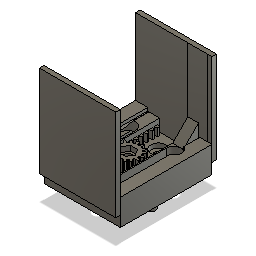
Spool Saver (Autodesk Fusion 360 design; units mm, degrees)
description: Spur Gear; Module: 1.000000; Num Teeth: 16; Pressure Angle: 20.000000; Backlash: 0.05 mm
Autodesk Fusion 360 part; units mm, degrees
(part 1 of 5)
sketch "Side Profile" plane through (0, 0, 0) normal (0, 0, 1) x (1, 0, 0)
  line L0 (0, 0) -> (25, 0)
  line L1 (25, 7) -> (3, 7)
  line L2 (8, 17.2) -> (0, 17.2)
  line L3 (0, 17.2) -> (0, 0)
  line L4 (8, 17.2) -> (8, 15.2)
  line L5 (3, 7) -> (3, 8.0593)
  line L6 (3, 8.0593) -> (8, 15.2)
  line L7 (50, 17.2) -> (50, 0)
  line L8 (50, 0) -> (25, 0)
  line L9 (47, 7) -> (47, 8.0593)
  line L10 (42, 17.2) -> (50, 17.2)
  line L11 (47, 8.0593) -> (42, 15.2)
  line L12 (25, 7) -> (47, 7)
  line L13 (42, 17.2) -> (42, 15.2)
  point P0 (50, 0)
  dimension "d2" = 7
  dimension "d3" = 17.2
  dimension "d4" = 8
  dimension "d5" = 2
  dimension "d8" = 22
  dimension "d9" = 145
  constraint coincident L0.start L3.end
  constraint horizontal L0
  constraint perpendicular L0 L3
  constraint perpendicular L2 L4
  constraint perpendicular L1 L5
  measures "d2" distance of L0.end L1.start
  measures "d3" distance of L0.start L2.end
  measures "d4" distance of L2.start L2.end
  measures "d5" distance of L2.start L4.end
  measures "d8" distance of L1.start L1.end
  measures "d9" angle of L4 L6
extrude "Extrude1" add sketch "Side Profile" along normal blind 60 makes body 1
sketch "Base Top" plane through (0, 7, 0) normal (0, 1, 0) x (-1, 0, 0)
  line L0 (-47, 0) -> (-3, 0)
  line L1 (-3, 0) -> (-3, 60)
  line L2 (-3, 60) -> (-47, 60)
  circle A0 centre (-25, 30) radius 4.475
  circle A1 centre (-25, 30) radius 2.6
  line L3 (0, 0) -> (0, 60)
  line L4 (-50, 0) -> (-50, 60)
  line L5 (0, 30) -> (-50, 30) construction
  circle A2 centre (-40, 15) radius 2.45
  line L6 (-3, 0) -> (-47, 0)
  line L7 (-50, 0) -> (-50, 60)
  circle A3 centre (-10, 45) radius 2.45
  circle A4 centre (-40, 15) radius 5
  circle A5 centre (-10, 45) radius 5
  line L8 (-47, 60) -> (-47, 0)
  line L9 (-47, 0) -> (-3, 0)
  line L10 (-3, 0) -> (-3, 60)
  line L11 (-3, 60) -> (-47, 60)
  line L12 (-47, 60) -> (-47, 0)
  line L13 (-37.55, 15) -> (-37.55, 3)
  line L14 (-42, 0) -> (-42, 60)
  line L15 (-42.45, 15) -> (-42.45, 3)
  line L16 (-37.55, 3) -> (-42.45, 3)
  line L17 (-12.45, 45) -> (-12.45, 57)
  line L18 (-8, 0) -> (-8, 60)
  line L19 (-7.55, 45) -> (-7.55, 57)
  line L20 (-12.45, 57) -> (-7.55, 57)
  circle A6 centre (-25, 10) radius 2.6
  circle A7 centre (-25, 10) radius 5
  line L21 (0, 0) -> (0, 60)
  circle A8 centre (-25, 50) radius 2.6
  circle A9 centre (-25, 50) radius 5
  dimension "d14" = 8.95
  dimension "d15" = 5.2
  dimension "d20" = 4.9
  dimension "d21" = 15
  dimension "d22" = 10
  dimension "d24" = 10
  dimension "d25" = 10
  dimension "d26" = 15
  dimension "d46" = 12
  dimension "d115" = 5.2
  dimension "d116" = 10
  dimension "d117" = 10
  dimension "d118" = 25
  constraint coincident A0.centre A1.centre
  constraint midpoint L3 L5.start
  constraint midpoint L4 L5.end
  constraint equal A2 A3
  constraint concentric A2 A4
  constraint concentric A3 A5
  constraint equal A4 A5
  constraint vertical L13
  constraint parallel L14 L15
  constraint equal L13 L15
  constraint tangent A2 L13
  constraint tangent A2 L15
  constraint coincident A2 L13.start
  constraint coincident A2 L15.start
  constraint coincident A3 L17.start
  constraint coincident A3 L19.start
  constraint parallel L18 L19
  constraint equal L13 L17
  constraint equal L15 L19
  constraint equal L16 L20
  constraint concentric A6 A7
  constraint symmetric L5 A6 A8
  constraint symmetric L5 A7 A9
  measures "d14" diameter of A0
  measures "d15" diameter of A1
  measures "d20" diameter of A2
  measures "d21" distance of A2.centre L6
  measures "d22" distance of A2.centre L7
  measures "d24" diameter of A4
  measures "d25" distance of L3 A3.centre
  measures "d26" distance of L2 A3.centre
  measures "d46" distance of L13.start L13.end
  measures "d115" diameter of A6
  measures "d116" diameter of A7
  measures "d117" distance of L6 A6.centre
  measures "d118" distance of A6.centre L21
extrude "Extrude4" cut sketch "Base Top" against normal up to surface (7 mm away) contours A3 L18 | A3 L18 | A2 L14 | A2 L14 | A1 bodies 1
extrude "Extrude5" add sketch "Base Top" along normal blind 2.5 contours A0 bodies 1
sketch "Sketch1" plane through (0, 0, 0) normal (0, 0, 1) x (1, 0, 0) in component "Spur Gear (16 teeth)"
  circle A0 centre (0, 0) radius 6.7492
  circle A1 centre (0, 0) radius 2.5
extrude "Extrude1'" add sketch "Sketch1" along normal blind 5 separate body makes body 2 in component "Spur Gear (16 teeth)"
sketch "Sketch2" plane through (0, 0, 0) normal (0, 0, 1) x (1, 0, 0) in component "Spur Gear (16 teeth)"
  spline S0 degree 5 poles (7.4708, -0.8366) (7.4752, -0.8371) (7.4838, -0.8379) (7.4968, -0.8388) (7.5141, -0.8393) (7.5358, -0.8389) (7.5576, -0.8379) (7.5793, -0.8364) (7.6012, -0.8347) (7.623, -0.8328) (7.6449, -0.8308) (7.6667, -0.8285) (7.6886, -0.826) (7.7105, -0.8231) (7.7325, -0.8199) (7.7544, -0.8163) (7.7763, -0.8125) (7.7983, -0.8084) (7.8202, -0.8042) (7.8422, -0.7997) (7.8641, -0.7951) (7.8861, -0.7903) (7.9081, -0.7852) (7.93, -0.78) (7.952, -0.7745) (7.974, -0.7688) (7.9959, -0.763) (8.0179, -0.7569) (8.0399, -0.7506) (8.0618, -0.7442) (8.0838, -0.7376) (8.1057, -0.7308) (8.1277, -0.7239) (8.1496, -0.7168) (8.1716, -0.7095) (8.1935, -0.702) (8.2154, -0.6944) (8.2373, -0.6865) (8.2592, -0.6786) (8.2811, -0.6704) (8.303, -0.6622) (8.3248, -0.6537) (8.3467, -0.6451) (8.3685, -0.6363) (8.3904, -0.6274) (8.4122, -0.6183) (8.434, -0.6091) (8.4558, -0.5997) (8.4776, -0.5902) (8.4993, -0.5805) (8.5211, -0.5707) (8.5428, -0.5607) (8.5645, -0.5506) (8.5862, -0.5403) (8.6079, -0.5299) (8.6295, -0.5193) (8.6511, -0.5086) (8.6728, -0.4978) (8.6944, -0.4868) (8.7159, -0.4757) (8.7375, -0.4644) (8.759, -0.453) (8.7805, -0.4415) (8.802, -0.4298) (8.8235, -0.418) (8.8449, -0.4061) (8.8664, -0.394) (8.8878, -0.3818) (8.9091, -0.3695) (8.9305, -0.357) (8.9518, -0.3444) (8.9688, -0.3342) (8.9816, -0.3265) (8.9901, -0.3213) (8.9944, -0.3187) knots 0 0 0 0 0 0 0.01428571 0.02857143 0.04285714 0.05714286 0.07142857 0.08571429 0.1 0.11428571 0.12857143 0.14285714 0.15714286 0.17142857 0.18571429 0.2 0.21428571 0.22857143 0.24285714 0.25714286 0.27142857 0.28571429 0.3 0.31428571 0.32857143 0.34285714 0.35714286 0.37142857 0.38571429 0.4 0.41428571 0.42857143 0.44285714 0.45714286 0.47142857 0.48571429 0.5 0.51428571 0.52857143 0.54285714 0.55714286 0.57142857 0.58571429 0.6 0.61428571 0.62857143 0.64285714 0.65714286 0.67142857 0.68571429 0.7 0.71428571 0.72857143 0.74285714 0.75714286 0.77142857 0.78571429 0.8 0.81428571 0.82857143 0.84285714 0.85714286 0.87142857 0.88571429 0.9 0.91428571 0.92857143 0.94285714 0.95714286 0.97142857 0.98571429 1 1 1 1 1 1
  spline S1 degree 5 poles (7.4708, 0.8366) (7.4752, 0.8371) (7.4838, 0.8379) (7.4968, 0.8388) (7.5141, 0.8393) (7.5358, 0.8389) (7.5576, 0.8379) (7.5793, 0.8364) (7.6012, 0.8347) (7.623, 0.8328) (7.6449, 0.8308) (7.6667, 0.8285) (7.6886, 0.826) (7.7105, 0.8231) (7.7325, 0.8199) (7.7544, 0.8163) (7.7763, 0.8125) (7.7983, 0.8084) (7.8202, 0.8042) (7.8422, 0.7997) (7.8641, 0.7951) (7.8861, 0.7903) (7.9081, 0.7852) (7.93, 0.78) (7.952, 0.7745) (7.974, 0.7688) (7.9959, 0.763) (8.0179, 0.7569) (8.0399, 0.7506) (8.0618, 0.7442) (8.0838, 0.7376) (8.1057, 0.7308) (8.1277, 0.7239) (8.1496, 0.7168) (8.1716, 0.7095) (8.1935, 0.702) (8.2154, 0.6944) (8.2373, 0.6865) (8.2592, 0.6786) (8.2811, 0.6704) (8.303, 0.6622) (8.3248, 0.6537) (8.3467, 0.6451) (8.3685, 0.6363) (8.3904, 0.6274) (8.4122, 0.6183) (8.434, 0.6091) (8.4558, 0.5997) (8.4776, 0.5902) (8.4993, 0.5805) (8.5211, 0.5707) (8.5428, 0.5607) (8.5645, 0.5506) (8.5862, 0.5403) (8.6079, 0.5299) (8.6295, 0.5193) (8.6511, 0.5086) (8.6728, 0.4978) (8.6944, 0.4868) (8.7159, 0.4757) (8.7375, 0.4644) (8.759, 0.453) (8.7805, 0.4415) (8.802, 0.4298) (8.8235, 0.418) (8.8449, 0.4061) (8.8664, 0.394) (8.8878, 0.3818) (8.9091, 0.3695) (8.9305, 0.357) (8.9518, 0.3444) (8.9688, 0.3342) (8.9816, 0.3265) (8.9901, 0.3213) (8.9944, 0.3187) knots 0 0 0 0 0 0 0.01428571 0.02857143 0.04285714 0.05714286 0.07142857 0.08571429 0.1 0.11428571 0.12857143 0.14285714 0.15714286 0.17142857 0.18571429 0.2 0.21428571 0.22857143 0.24285714 0.25714286 0.27142857 0.28571429 0.3 0.31428571 0.32857143 0.34285714 0.35714286 0.37142857 0.38571429 0.4 0.41428571 0.42857143 0.44285714 0.45714286 0.47142857 0.48571429 0.5 0.51428571 0.52857143 0.54285714 0.55714286 0.57142857 0.58571429 0.6 0.61428571 0.62857143 0.64285714 0.65714286 0.67142857 0.68571429 0.7 0.71428571 0.72857143 0.74285714 0.75714286 0.77142857 0.78571429 0.8 0.81428571 0.82857143 0.84285714 0.85714286 0.87142857 0.88571429 0.9 0.91428571 0.92857143 0.94285714 0.95714286 0.97142857 0.98571429 1 1 1 1 1 1
  arc A0 (8.9944, -0.3187) -> (8.9944, 0.3187) centre (0, 0) ccw
  line L0 (6.6973, -0.7511) -> (7.4708, -0.8366)
  line L1 (6.6973, 0.7511) -> (7.4708, 0.8366)
  line L2 (6.6973, -0.7511) -> (6.6973, 0.7511)
  point P0 (7.5774, -0.8365)
  point P1 (7.685, -0.8263)
  point P2 (7.7933, -0.8093)
  point P3 (7.902, -0.7866)
  point P4 (8.0111, -0.7587)
  point P5 (8.1205, -0.7262)
  point P6 (8.23, -0.6891)
  point P7 (8.3395, -0.6479)
  point P8 (8.4491, -0.6026)
  point P9 (8.5586, -0.5533)
  point P10 (8.6679, -0.5002)
  point P11 (8.777, -0.4434)
  point P12 (8.8859, -0.3828)
  point P13 (7.5774, 0.8365)
  point P14 (7.685, 0.8263)
  point P15 (7.7933, 0.8093)
  point P16 (7.902, 0.7866)
  point P17 (8.0111, 0.7587)
  point P18 (8.1205, 0.7262)
  point P19 (8.23, 0.6891)
  point P20 (8.3395, 0.6479)
  point P21 (8.4491, 0.6026)
  point P22 (8.5586, 0.5533)
  point P23 (8.6679, 0.5002)
  point P24 (8.777, 0.4434)
  point P25 (8.8859, 0.3828)
extrude "Extrude2" add sketch "Sketch2" along normal blind 5 bodies 2 in component "Spur Gear (16 teeth)"
fillet "Fillet1" radius 0.5 2 edges at (6.7072, -0.7522, 2.5) (6.7072, 0.7522, 2.5) on bodies 2 in component "Spur Gear (16 teeth)"
pattern_circular "C-Pattern1" count 16 over 360 about axis through (0, 0, 0) along (0, 0, 1) of "Extrude2", "Fillet1" in component "Spur Gear (16 teeth)"
sketch "Sketch3" plane through (0, 0, 0) normal (0, 0, 1) x (1, 0, 0) in component "Spur Gear (16 teeth)"
  circle A0 centre (0, 0) radius 8 construction
move_body "Move1" bodies 2 to x (1, 0, 0) y (0, 1, 0) z (0, 0, 1) at (25, 7, 30) in component "Spur Gear (16 teeth)"
move_body "Move2" bodies 2 to x (1, 0, 0) y (0, 0, -1) z (0, 1, 0) at (0, -23, 37) in component "Spur Gear (16 teeth)"
move_body "Move3" bodies 2 to x (0.980785, 0, -0.19509) y (0, 1, 0) z (0.19509, 0, 0.980785) at (-5.3723, 0, 5.4537) in component "Spur Gear (16 teeth)"
cylinder "CylinderPrimitive1" add diameter 5 height -2.5 placed x (1, 0, 0) y (0, 0, -1) z (0, 1, 0) at (25, 12, 30) bodies 2 in component "Spur Gear (16 teeth)"
extrude "Extrude3" add 1 faces at (22.1207, 12, 28.6457) along direction (0, 1, 0) blind 4 on bodies 2 bodies 2 in component "Spur Gear (16 teeth)"
sketch "Nut and Hole" plane through (0, 16, 0) normal (0, 1, 0) x (-1, 0, 0) in component "Spur Gear (16 teeth)"
  arc A0 (-31.7484, 30.1063) -> (-31.7484, 29.8937) centre (-25, 30) ccw
  arc A1 (-32.2052, 29.3877) -> (-31.7484, 29.8937) centre (-32.2483, 29.8858) ccw
  line L0 (-32.2052, 29.3877) -> (-32.4905, 29.363)
  spline S0 degree 5 poles (-32.4905, 29.363) (-32.4948, 29.3627) (-32.5035, 29.3618) (-32.5163, 29.3601) (-32.5334, 29.3572) (-32.5547, 29.3527) (-32.5758, 29.3474) (-32.5969, 29.3417) (-32.618, 29.3358) (-32.639, 29.3297) (-32.6601, 29.3234) (-32.6811, 29.3169) (-32.702, 29.3101) (-32.723, 29.303) (-32.7438, 29.2956) (-32.7646, 29.2878) (-32.7854, 29.2798) (-32.8061, 29.2715) (-32.8269, 29.2631) (-32.8475, 29.2544) (-32.8682, 29.2456) (-32.8888, 29.2366) (-32.9093, 29.2274) (-32.9298, 29.2179) (-32.9503, 29.2083) (-32.9707, 29.1984) (-32.9911, 29.1884) (-33.0115, 29.1781) (-33.0318, 29.1677) (-33.0521, 29.1571) (-33.0724, 29.1464) (-33.0926, 29.1355) (-33.1127, 29.1244) (-33.1329, 29.1131) (-33.1529, 29.1016) (-33.173, 29.09) (-33.193, 29.0783) (-33.213, 29.0663) (-33.2329, 29.0542) (-33.2528, 29.042) (-33.2726, 29.0296) (-33.2924, 29.017) (-33.3122, 29.0043) (-33.3319, 28.9915) (-33.3515, 28.9785) (-33.3712, 28.9653) (-33.3908, 28.952) (-33.4103, 28.9385) (-33.4298, 28.925) (-33.4492, 28.9112) (-33.4687, 28.8973) (-33.488, 28.8833) (-33.5073, 28.8691) (-33.5266, 28.8548) (-33.5458, 28.8404) (-33.565, 28.8258) (-33.5841, 28.8111) (-33.6032, 28.7963) (-33.6223, 28.7813) (-33.6413, 28.7662) (-33.6602, 28.7509) (-33.6791, 28.7355) (-33.698, 28.72) (-33.7168, 28.7044) (-33.7355, 28.6886) (-33.7542, 28.6727) (-33.7729, 28.6567) (-33.7915, 28.6405) (-33.81, 28.6243) (-33.8285, 28.6079) (-33.847, 28.5913) (-33.8617, 28.578) (-33.8727, 28.568) (-33.88, 28.5613) (-33.8837, 28.5579) knots 0 0 0 0 0 0 0.01428571 0.02857143 0.04285714 0.05714286 0.07142857 0.08571429 0.1 0.11428571 0.12857143 0.14285714 0.15714286 0.17142857 0.18571429 0.2 0.21428571 0.22857143 0.24285714 0.25714286 0.27142857 0.28571429 0.3 0.31428571 0.32857143 0.34285714 0.35714286 0.37142857 0.38571429 0.4 0.41428571 0.42857143 0.44285714 0.45714286 0.47142857 0.48571429 0.5 0.51428571 0.52857143 0.54285714 0.55714286 0.57142857 0.58571429 0.6 0.61428571 0.62857143 0.64285714 0.65714286 0.67142857 0.68571429 0.7 0.71428571 0.72857143 0.74285714 0.75714286 0.77142857 0.78571429 0.8 0.81428571 0.82857143 0.84285714 0.85714286 0.87142857 0.88571429 0.9 0.91428571 0.92857143 0.94285714 0.95714286 0.97142857 0.98571429 1 1 1 1 1 1
  arc A2 (-33.8837, 28.5579) -> (-33.7594, 27.9327) centre (-25, 30) ccw
  spline S1 degree 5 poles (-33.7594, 27.9327) (-33.7547, 27.931) (-33.7453, 27.9276) (-33.7313, 27.9225) (-33.7126, 27.9158) (-33.6892, 27.9076) (-33.6659, 27.8996) (-33.6425, 27.8916) (-33.6191, 27.8838) (-33.5958, 27.8762) (-33.5724, 27.8686) (-33.549, 27.8612) (-33.5257, 27.854) (-33.5023, 27.8469) (-33.479, 27.8399) (-33.4557, 27.833) (-33.4323, 27.8264) (-33.409, 27.8198) (-33.3857, 27.8134) (-33.3624, 27.8071) (-33.3391, 27.801) (-33.3158, 27.795) (-33.2925, 27.7892) (-33.2692, 27.7835) (-33.246, 27.7779) (-33.2227, 27.7725) (-33.1995, 27.7673) (-33.1763, 27.7622) (-33.1531, 27.7572) (-33.1299, 27.7524) (-33.1067, 27.7478) (-33.0836, 27.7433) (-33.0605, 27.7389) (-33.0373, 27.7348) (-33.0142, 27.7307) (-32.9912, 27.7269) (-32.9681, 27.7232) (-32.9451, 27.7196) (-32.9221, 27.7162) (-32.8991, 27.713) (-32.8761, 27.71) (-32.8532, 27.7071) (-32.8303, 27.7044) (-32.8074, 27.7018) (-32.7846, 27.6995) (-32.7617, 27.6973) (-32.7389, 27.6953) (-32.7162, 27.6934) (-32.6935, 27.6918) (-32.6708, 27.6903) (-32.6481, 27.689) (-32.6255, 27.6879) (-32.6029, 27.6871) (-32.5804, 27.6864) (-32.5579, 27.6859) (-32.5355, 27.6857) (-32.5131, 27.6856) (-32.4907, 27.6857) (-32.4684, 27.686) (-32.4461, 27.6866) (-32.4239, 27.6874) (-32.4018, 27.6885) (-32.3798, 27.6899) (-32.3578, 27.6917) (-32.3359, 27.6937) (-32.3141, 27.696) (-32.2923, 27.6984) (-32.2705, 27.701) (-32.2489, 27.7038) (-32.2273, 27.707) (-32.206, 27.7109) (-32.1891, 27.7148) (-32.1765, 27.7182) (-32.1682, 27.7207) (-32.1641, 27.722) knots -1 -1 -1 -1 -1 -1 -0.98571429 -0.97142857 -0.95714286 -0.94285714 -0.92857143 -0.91428571 -0.9 -0.88571429 -0.87142857 -0.85714286 -0.84285714 -0.82857143 -0.81428571 -0.8 -0.78571429 -0.77142857 -0.75714286 -0.74285714 -0.72857143 -0.71428571 -0.7 -0.68571429 -0.67142857 -0.65714286 -0.64285714 -0.62857143 -0.61428571 -0.6 -0.58571429 -0.57142857 -0.55714286 -0.54285714 -0.52857143 -0.51428571 -0.5 -0.48571429 -0.47142857 -0.45714286 -0.44285714 -0.42857143 -0.41428571 -0.4 -0.38571429 -0.37142857 -0.35714286 -0.34285714 -0.32857143 -0.31428571 -0.3 -0.28571429 -0.27142857 -0.25714286 -0.24285714 -0.22857143 -0.21428571 -0.2 -0.18571429 -0.17142857 -0.15714286 -0.14285714 -0.12857143 -0.11428571 -0.1 -0.08571429 -0.07142857 -0.05714286 -0.04285714 -0.02857143 -0.01428571 0 0 0 0 0 0
  line L1 (-32.1641, 27.722) -> (-31.8911, 27.8084)
  arc A3 (-31.2753, 27.5157) -> (-31.8911, 27.8084) centre (-31.7402, 27.3317) ccw
  arc A4 (-31.2753, 27.5157) -> (-31.194, 27.3193) centre (-25, 30) ccw
  arc A5 (-31.4224, 26.677) -> (-31.194, 27.3193) centre (-31.6529, 27.1207) ccw
  line L2 (-31.4224, 26.677) -> (-31.6766, 26.545)
  spline S2 degree 5 poles (-31.6766, 26.545) (-31.6804, 26.543) (-31.6881, 26.5389) (-31.6993, 26.5325) (-31.714, 26.5232) (-31.7319, 26.5109) (-31.7494, 26.4979) (-31.7667, 26.4846) (-31.7839, 26.4711) (-31.801, 26.4574) (-31.818, 26.4435) (-31.835, 26.4295) (-31.8518, 26.4152) (-31.8684, 26.4006) (-31.8848, 26.3858) (-31.9011, 26.3706) (-31.9172, 26.3553) (-31.9332, 26.3397) (-31.9491, 26.324) (-31.9649, 26.3081) (-31.9805, 26.292) (-31.9961, 26.2758) (-32.0116, 26.2594) (-32.0269, 26.2428) (-32.0421, 26.2261) (-32.0573, 26.2092) (-32.0723, 26.1921) (-32.0872, 26.1748) (-32.1019, 26.1574) (-32.1166, 26.1399) (-32.1312, 26.1222) (-32.1457, 26.1044) (-32.1601, 26.0864) (-32.1744, 26.0683) (-32.1886, 26.05) (-32.2026, 26.0316) (-32.2166, 26.0131) (-32.2305, 25.9944) (-32.2443, 25.9756) (-32.258, 25.9567) (-32.2715, 25.9377) (-32.285, 25.9185) (-32.2984, 25.8992) (-32.3117, 25.8798) (-32.3249, 25.8602) (-32.338, 25.8406) (-32.351, 25.8208) (-32.3639, 25.8009) (-32.3767, 25.7808) (-32.3894, 25.7607) (-32.402, 25.7405) (-32.4146, 25.7201) (-32.427, 25.6996) (-32.4393, 25.679) (-32.4516, 25.6583) (-32.4637, 25.6375) (-32.4757, 25.6166) (-32.4877, 25.5956) (-32.4996, 25.5744) (-32.5113, 25.5532) (-32.523, 25.5319) (-32.5346, 25.5104) (-32.546, 25.4889) (-32.5574, 25.4672) (-32.5687, 25.4455) (-32.5799, 25.4237) (-32.591, 25.4017) (-32.602, 25.3797) (-32.6129, 25.3575) (-32.6237, 25.3353) (-32.6345, 25.313) (-32.643, 25.295) (-32.6493, 25.2815) (-32.6535, 25.2725) (-32.6556, 25.268) knots 0 0 0 0 0 0 0.01428571 0.02857143 0.04285714 0.05714286 0.07142857 0.08571429 0.1 0.11428571 0.12857143 0.14285714 0.15714286 0.17142857 0.18571429 0.2 0.21428571 0.22857143 0.24285714 0.25714286 0.27142857 0.28571429 0.3 0.31428571 0.32857143 0.34285714 0.35714286 0.37142857 0.38571429 0.4 0.41428571 0.42857143 0.44285714 0.45714286 0.47142857 0.48571429 0.5 0.51428571 0.52857143 0.54285714 0.55714286 0.57142857 0.58571429 0.6 0.61428571 0.62857143 0.64285714 0.65714286 0.67142857 0.68571429 0.7 0.71428571 0.72857143 0.74285714 0.75714286 0.77142857 0.78571429 0.8 0.81428571 0.82857143 0.84285714 0.85714286 0.87142857 0.88571429 0.9 0.91428571 0.92857143 0.94285714 0.95714286 0.97142857 0.98571429 1 1 1 1 1 1
  arc A6 (-32.6556, 25.268) -> (-32.3015, 24.738) centre (-25, 30) ccw
  spline S3 degree 5 poles (-32.3015, 24.738) (-32.2965, 24.7382) (-32.2865, 24.7386) (-32.2717, 24.7393) (-32.2518, 24.7403) (-32.2271, 24.7417) (-32.2024, 24.7432) (-32.1778, 24.7448) (-32.1532, 24.7465) (-32.1287, 24.7484) (-32.1042, 24.7503) (-32.0798, 24.7525) (-32.0555, 24.7547) (-32.0312, 24.7571) (-32.0069, 24.7595) (-31.9828, 24.7622) (-31.9586, 24.7649) (-31.9346, 24.7678) (-31.9106, 24.7708) (-31.8866, 24.7739) (-31.8628, 24.7771) (-31.839, 24.7805) (-31.8152, 24.784) (-31.7916, 24.7877) (-31.7679, 24.7915) (-31.7444, 24.7954) (-31.7209, 24.7994) (-31.6975, 24.8036) (-31.6742, 24.8079) (-31.651, 24.8123) (-31.6278, 24.8169) (-31.6047, 24.8216) (-31.5816, 24.8265) (-31.5587, 24.8314) (-31.5358, 24.8366) (-31.513, 24.8418) (-31.4903, 24.8472) (-31.4676, 24.8528) (-31.4451, 24.8584) (-31.4226, 24.8643) (-31.4002, 24.8702) (-31.3779, 24.8763) (-31.3557, 24.8826) (-31.3336, 24.889) (-31.3116, 24.8956) (-31.2897, 24.9023) (-31.2679, 24.9091) (-31.2461, 24.9162) (-31.2245, 24.9233) (-31.203, 24.9306) (-31.1816, 24.9381) (-31.1603, 24.9458) (-31.1391, 24.9536) (-31.118, 24.9616) (-31.0971, 24.9698) (-31.0762, 24.9782) (-31.0555, 24.9867) (-31.0349, 24.9953) (-31.0144, 25.0041) (-30.994, 25.0132) (-30.9738, 25.0224) (-30.9538, 25.0319) (-30.934, 25.0417) (-30.9144, 25.0517) (-30.8949, 25.062) (-30.8756, 25.0724) (-30.8564, 25.083) (-30.8373, 25.0937) (-30.8184, 25.1046) (-30.7997, 25.1158) (-30.7814, 25.1276) (-30.7673, 25.1376) (-30.757, 25.1455) (-30.7503, 25.151) (-30.747, 25.1538) knots -1 -1 -1 -1 -1 -1 -0.98571429 -0.97142857 -0.95714286 -0.94285714 -0.92857143 -0.91428571 -0.9 -0.88571429 -0.87142857 -0.85714286 -0.84285714 -0.82857143 -0.81428571 -0.8 -0.78571429 -0.77142857 -0.75714286 -0.74285714 -0.72857143 -0.71428571 -0.7 -0.68571429 -0.67142857 -0.65714286 -0.64285714 -0.62857143 -0.61428571 -0.6 -0.58571429 -0.57142857 -0.55714286 -0.54285714 -0.52857143 -0.51428571 -0.5 -0.48571429 -0.47142857 -0.45714286 -0.44285714 -0.42857143 -0.41428571 -0.4 -0.38571429 -0.37142857 -0.35714286 -0.34285714 -0.32857143 -0.31428571 -0.3 -0.28571429 -0.27142857 -0.25714286 -0.24285714 -0.22857143 -0.21428571 -0.2 -0.18571429 -0.17142857 -0.15714286 -0.14285714 -0.12857143 -0.11428571 -0.1 -0.08571429 -0.07142857 -0.05714286 -0.04285714 -0.02857143 -0.01428571 0 0 0 0 0 0
  line L3 (-30.747, 25.1538) -> (-30.5278, 25.3381)
  arc A7 (-29.847, 25.3033) -> (-30.5278, 25.3381) centre (-30.206, 24.9554) ccw
  arc A8 (-29.847, 25.3033) -> (-29.6967, 25.153) centre (-25, 30) ccw
  arc A9 (-29.6619, 24.4722) -> (-29.6967, 25.153) centre (-30.0446, 24.794) ccw
  line L4 (-29.6619, 24.4722) -> (-29.8462, 24.253)
  spline S4 degree 5 poles (-29.8462, 24.253) (-29.849, 24.2497) (-29.8545, 24.243) (-29.8624, 24.2327) (-29.8724, 24.2186) (-29.8842, 24.2003) (-29.8954, 24.1816) (-29.9063, 24.1627) (-29.917, 24.1436) (-29.9276, 24.1244) (-29.938, 24.1051) (-29.9483, 24.0856) (-29.9583, 24.066) (-29.9681, 24.0462) (-29.9776, 24.0262) (-29.9868, 24.006) (-29.9959, 23.9856) (-30.0047, 23.9651) (-30.0133, 23.9445) (-30.0218, 23.9238) (-30.0302, 23.9029) (-30.0384, 23.882) (-30.0464, 23.8609) (-30.0542, 23.8397) (-30.0619, 23.8184) (-30.0694, 23.797) (-30.0767, 23.7755) (-30.0838, 23.7539) (-30.0909, 23.7321) (-30.0977, 23.7103) (-30.1044, 23.6884) (-30.111, 23.6664) (-30.1174, 23.6443) (-30.1237, 23.6221) (-30.1298, 23.5998) (-30.1357, 23.5774) (-30.1416, 23.5549) (-30.1472, 23.5324) (-30.1528, 23.5097) (-30.1582, 23.487) (-30.1634, 23.4642) (-30.1686, 23.4413) (-30.1735, 23.4184) (-30.1784, 23.3953) (-30.1831, 23.3722) (-30.1877, 23.349) (-30.1921, 23.3258) (-30.1964, 23.3025) (-30.2006, 23.2791) (-30.2046, 23.2556) (-30.2085, 23.2321) (-30.2123, 23.2084) (-30.216, 23.1848) (-30.2195, 23.161) (-30.2229, 23.1372) (-30.2261, 23.1134) (-30.2292, 23.0894) (-30.2322, 23.0654) (-30.2351, 23.0414) (-30.2378, 23.0172) (-30.2405, 22.9931) (-30.2429, 22.9688) (-30.2453, 22.9445) (-30.2475, 22.9202) (-30.2497, 22.8958) (-30.2516, 22.8713) (-30.2535, 22.8468) (-30.2552, 22.8222) (-30.2568, 22.7976) (-30.2583, 22.7729) (-30.2597, 22.7482) (-30.2607, 22.7283) (-30.2614, 22.7135) (-30.2618, 22.7035) (-30.262, 22.6985) knots 0 0 0 0 0 0 0.01428571 0.02857143 0.04285714 0.05714286 0.07142857 0.08571429 0.1 0.11428571 0.12857143 0.14285714 0.15714286 0.17142857 0.18571429 0.2 0.21428571 0.22857143 0.24285714 0.25714286 0.27142857 0.28571429 0.3 0.31428571 0.32857143 0.34285714 0.35714286 0.37142857 0.38571429 0.4 0.41428571 0.42857143 0.44285714 0.45714286 0.47142857 0.48571429 0.5 0.51428571 0.52857143 0.54285714 0.55714286 0.57142857 0.58571429 0.6 0.61428571 0.62857143 0.64285714 0.65714286 0.67142857 0.68571429 0.7 0.71428571 0.72857143 0.74285714 0.75714286 0.77142857 0.78571429 0.8 0.81428571 0.82857143 0.84285714 0.85714286 0.87142857 0.88571429 0.9 0.91428571 0.92857143 0.94285714 0.95714286 0.97142857 0.98571429 1 1 1 1 1 1
  arc A10 (-30.262, 22.6985) -> (-29.732, 22.3444) centre (-25, 30) ccw
  spline S5 degree 5 poles (-29.732, 22.3444) (-29.7275, 22.3465) (-29.7185, 22.3507) (-29.705, 22.357) (-29.687, 22.3655) (-29.6647, 22.3763) (-29.6425, 22.3871) (-29.6203, 22.398) (-29.5983, 22.409) (-29.5763, 22.4201) (-29.5545, 22.4313) (-29.5328, 22.4426) (-29.5111, 22.454) (-29.4896, 22.4654) (-29.4681, 22.477) (-29.4468, 22.4887) (-29.4256, 22.5004) (-29.4044, 22.5123) (-29.3834, 22.5243) (-29.3625, 22.5363) (-29.3417, 22.5484) (-29.321, 22.5607) (-29.3004, 22.573) (-29.2799, 22.5854) (-29.2595, 22.598) (-29.2393, 22.6106) (-29.2192, 22.6233) (-29.1991, 22.6361) (-29.1792, 22.649) (-29.1594, 22.662) (-29.1398, 22.6751) (-29.1202, 22.6883) (-29.1008, 22.7016) (-29.0815, 22.715) (-29.0623, 22.7285) (-29.0433, 22.742) (-29.0244, 22.7557) (-29.0056, 22.7695) (-28.9869, 22.7834) (-28.9684, 22.7974) (-28.95, 22.8114) (-28.9317, 22.8256) (-28.9136, 22.8399) (-28.8956, 22.8543) (-28.8778, 22.8688) (-28.8601, 22.8834) (-28.8426, 22.8981) (-28.8252, 22.9128) (-28.8079, 22.9277) (-28.7908, 22.9427) (-28.7739, 22.9579) (-28.7572, 22.9731) (-28.7406, 22.9884) (-28.7242, 23.0039) (-28.708, 23.0195) (-28.6919, 23.0351) (-28.676, 23.0509) (-28.6603, 23.0668) (-28.6447, 23.0828) (-28.6294, 23.0989) (-28.6142, 23.1152) (-28.5994, 23.1316) (-28.5848, 23.1482) (-28.5705, 23.165) (-28.5565, 23.182) (-28.5426, 23.199) (-28.5289, 23.2161) (-28.5154, 23.2333) (-28.5021, 23.2506) (-28.4891, 23.2681) (-28.4768, 23.286) (-28.4675, 23.3007) (-28.4611, 23.3119) (-28.457, 23.3196) (-28.455, 23.3234) knots -1 -1 -1 -1 -1 -1 -0.98571429 -0.97142857 -0.95714286 -0.94285714 -0.92857143 -0.91428571 -0.9 -0.88571429 -0.87142857 -0.85714286 -0.84285714 -0.82857143 -0.81428571 -0.8 -0.78571429 -0.77142857 -0.75714286 -0.74285714 -0.72857143 -0.71428571 -0.7 -0.68571429 -0.67142857 -0.65714286 -0.64285714 -0.62857143 -0.61428571 -0.6 -0.58571429 -0.57142857 -0.55714286 -0.54285714 -0.52857143 -0.51428571 -0.5 -0.48571429 -0.47142857 -0.45714286 -0.44285714 -0.42857143 -0.41428571 -0.4 -0.38571429 -0.37142857 -0.35714286 -0.34285714 -0.32857143 -0.31428571 -0.3 -0.28571429 -0.27142857 -0.25714286 -0.24285714 -0.22857143 -0.21428571 -0.2 -0.18571429 -0.17142857 -0.15714286 -0.14285714 -0.12857143 -0.11428571 -0.1 -0.08571429 -0.07142857 -0.05714286 -0.04285714 -0.02857143 -0.01428571 0 0 0 0 0 0
  line L5 (-28.455, 23.3234) -> (-28.323, 23.5776)
  arc A11 (-27.6807, 23.806) -> (-28.323, 23.5776) centre (-27.8793, 23.3471) ccw
  arc A12 (-27.6807, 23.806) -> (-27.4843, 23.7247) centre (-25, 30) ccw
  arc A13 (-27.1916, 23.1089) -> (-27.4843, 23.7247) centre (-27.6683, 23.2598) ccw
  line L6 (-27.1916, 23.1089) -> (-27.278, 22.8359)
  spline S6 degree 5 poles (-27.278, 22.8359) (-27.2793, 22.8318) (-27.2818, 22.8235) (-27.2852, 22.8109) (-27.2891, 22.794) (-27.293, 22.7727) (-27.2962, 22.7511) (-27.299, 22.7295) (-27.3016, 22.7077) (-27.304, 22.6859) (-27.3063, 22.6641) (-27.3083, 22.6422) (-27.3101, 22.6202) (-27.3115, 22.5982) (-27.3126, 22.5761) (-27.3134, 22.5539) (-27.314, 22.5316) (-27.3143, 22.5093) (-27.3144, 22.4869) (-27.3143, 22.4645) (-27.3141, 22.4421) (-27.3136, 22.4196) (-27.3129, 22.3971) (-27.3121, 22.3745) (-27.311, 22.3519) (-27.3097, 22.3292) (-27.3082, 22.3065) (-27.3066, 22.2838) (-27.3047, 22.2611) (-27.3027, 22.2383) (-27.3005, 22.2154) (-27.2982, 22.1926) (-27.2956, 22.1697) (-27.2929, 22.1468) (-27.29, 22.1239) (-27.287, 22.1009) (-27.2838, 22.0779) (-27.2804, 22.0549) (-27.2768, 22.0319) (-27.2731, 22.0088) (-27.2693, 21.9858) (-27.2652, 21.9627) (-27.2611, 21.9395) (-27.2567, 21.9164) (-27.2522, 21.8933) (-27.2476, 21.8701) (-27.2428, 21.8469) (-27.2378, 21.8237) (-27.2327, 21.8005) (-27.2275, 21.7773) (-27.2221, 21.754) (-27.2165, 21.7308) (-27.2108, 21.7075) (-27.205, 21.6842) (-27.199, 21.6609) (-27.1929, 21.6376) (-27.1866, 21.6143) (-27.1802, 21.591) (-27.1736, 21.5677) (-27.167, 21.5443) (-27.1601, 21.521) (-27.1531, 21.4977) (-27.146, 21.4743) (-27.1388, 21.451) (-27.1314, 21.4276) (-27.1238, 21.4042) (-27.1162, 21.3809) (-27.1084, 21.3575) (-27.1004, 21.3341) (-27.0924, 21.3108) (-27.0842, 21.2874) (-27.0775, 21.2687) (-27.0724, 21.2547) (-27.069, 21.2453) (-27.0673, 21.2406) knots 0 0 0 0 0 0 0.01428571 0.02857143 0.04285714 0.05714286 0.07142857 0.08571429 0.1 0.11428571 0.12857143 0.14285714 0.15714286 0.17142857 0.18571429 0.2 0.21428571 0.22857143 0.24285714 0.25714286 0.27142857 0.28571429 0.3 0.31428571 0.32857143 0.34285714 0.35714286 0.37142857 0.38571429 0.4 0.41428571 0.42857143 0.44285714 0.45714286 0.47142857 0.48571429 0.5 0.51428571 0.52857143 0.54285714 0.55714286 0.57142857 0.58571429 0.6 0.61428571 0.62857143 0.64285714 0.65714286 0.67142857 0.68571429 0.7 0.71428571 0.72857143 0.74285714 0.75714286 0.77142857 0.78571429 0.8 0.81428571 0.82857143 0.84285714 0.85714286 0.87142857 0.88571429 0.9 0.91428571 0.92857143 0.94285714 0.95714286 0.97142857 0.98571429 1 1 1 1 1 1
  arc A14 (-27.0673, 21.2406) -> (-26.4421, 21.1163) centre (-25, 30) ccw
  spline S7 degree 5 poles (-26.4421, 21.1163) (-26.4387, 21.12) (-26.432, 21.1273) (-26.422, 21.1383) (-26.4087, 21.153) (-26.3921, 21.1715) (-26.3757, 21.19) (-26.3595, 21.2085) (-26.3433, 21.2271) (-26.3273, 21.2458) (-26.3114, 21.2645) (-26.2956, 21.2832) (-26.28, 21.302) (-26.2645, 21.3209) (-26.2491, 21.3398) (-26.2338, 21.3587) (-26.2187, 21.3777) (-26.2037, 21.3968) (-26.1889, 21.4159) (-26.1742, 21.435) (-26.1596, 21.4542) (-26.1452, 21.4734) (-26.1309, 21.4927) (-26.1167, 21.512) (-26.1027, 21.5313) (-26.0888, 21.5508) (-26.075, 21.5702) (-26.0615, 21.5897) (-26.048, 21.6092) (-26.0347, 21.6288) (-26.0215, 21.6485) (-26.0085, 21.6681) (-25.9957, 21.6878) (-25.983, 21.7076) (-25.9704, 21.7274) (-25.958, 21.7472) (-25.9458, 21.7671) (-25.9337, 21.787) (-25.9217, 21.807) (-25.91, 21.827) (-25.8984, 21.8471) (-25.8869, 21.8671) (-25.8756, 21.8873) (-25.8645, 21.9074) (-25.8536, 21.9276) (-25.8429, 21.9479) (-25.8323, 21.9682) (-25.8219, 21.9885) (-25.8116, 22.0089) (-25.8016, 22.0293) (-25.7917, 22.0497) (-25.7821, 22.0702) (-25.7726, 22.0907) (-25.7634, 22.1112) (-25.7544, 22.1318) (-25.7456, 22.1525) (-25.7369, 22.1731) (-25.7285, 22.1939) (-25.7202, 22.2146) (-25.7122, 22.2354) (-25.7044, 22.2562) (-25.697, 22.277) (-25.6899, 22.298) (-25.6831, 22.3189) (-25.6766, 22.3399) (-25.6703, 22.361) (-25.6642, 22.382) (-25.6583, 22.4031) (-25.6526, 22.4242) (-25.6473, 22.4453) (-25.6428, 22.4666) (-25.6399, 22.4837) (-25.6382, 22.4965) (-25.6373, 22.5052) (-25.637, 22.5095) knots -1 -1 -1 -1 -1 -1 -0.98571429 -0.97142857 -0.95714286 -0.94285714 -0.92857143 -0.91428571 -0.9 -0.88571429 -0.87142857 -0.85714286 -0.84285714 -0.82857143 -0.81428571 -0.8 -0.78571429 -0.77142857 -0.75714286 -0.74285714 -0.72857143 -0.71428571 -0.7 -0.68571429 -0.67142857 -0.65714286 -0.64285714 -0.62857143 -0.61428571 -0.6 -0.58571429 -0.57142857 -0.55714286 -0.54285714 -0.52857143 -0.51428571 -0.5 -0.48571429 -0.47142857 -0.45714286 -0.44285714 -0.42857143 -0.41428571 -0.4 -0.38571429 -0.37142857 -0.35714286 -0.34285714 -0.32857143 -0.31428571 -0.3 -0.28571429 -0.27142857 -0.25714286 -0.24285714 -0.22857143 -0.21428571 -0.2 -0.18571429 -0.17142857 -0.15714286 -0.14285714 -0.12857143 -0.11428571 -0.1 -0.08571429 -0.07142857 -0.05714286 -0.04285714 -0.02857143 -0.01428571 0 0 0 0 0 0
  line L7 (-25.637, 22.5095) -> (-25.6123, 22.7948)
  arc A15 (-25.1063, 23.2516) -> (-25.6123, 22.7948) centre (-25.1142, 22.7517) ccw
  arc A16 (-25.1063, 23.2516) -> (-24.8937, 23.2516) centre (-25, 30) ccw
  arc A17 (-24.3877, 22.7948) -> (-24.8937, 23.2516) centre (-24.8858, 22.7517) ccw
  line L8 (-24.3877, 22.7948) -> (-24.363, 22.5095)
  spline S8 degree 5 poles (-24.363, 22.5095) (-24.3627, 22.5052) (-24.3618, 22.4965) (-24.3601, 22.4837) (-24.3572, 22.4666) (-24.3527, 22.4453) (-24.3474, 22.4242) (-24.3417, 22.4031) (-24.3358, 22.382) (-24.3297, 22.361) (-24.3234, 22.3399) (-24.3169, 22.3189) (-24.3101, 22.298) (-24.303, 22.277) (-24.2956, 22.2562) (-24.2878, 22.2354) (-24.2798, 22.2146) (-24.2715, 22.1939) (-24.2631, 22.1731) (-24.2544, 22.1525) (-24.2456, 22.1318) (-24.2366, 22.1112) (-24.2274, 22.0907) (-24.2179, 22.0702) (-24.2083, 22.0497) (-24.1984, 22.0293) (-24.1884, 22.0089) (-24.1781, 21.9885) (-24.1677, 21.9682) (-24.1571, 21.9479) (-24.1464, 21.9276) (-24.1355, 21.9074) (-24.1244, 21.8873) (-24.1131, 21.8671) (-24.1016, 21.8471) (-24.09, 21.827) (-24.0783, 21.807) (-24.0663, 21.787) (-24.0542, 21.7671) (-24.042, 21.7472) (-24.0296, 21.7274) (-24.017, 21.7076) (-24.0043, 21.6878) (-23.9915, 21.6681) (-23.9785, 21.6485) (-23.9653, 21.6288) (-23.952, 21.6092) (-23.9385, 21.5897) (-23.925, 21.5702) (-23.9112, 21.5508) (-23.8973, 21.5313) (-23.8833, 21.512) (-23.8691, 21.4927) (-23.8548, 21.4734) (-23.8404, 21.4542) (-23.8258, 21.435) (-23.8111, 21.4159) (-23.7963, 21.3968) (-23.7813, 21.3777) (-23.7662, 21.3587) (-23.7509, 21.3398) (-23.7355, 21.3209) (-23.72, 21.302) (-23.7044, 21.2832) (-23.6886, 21.2645) (-23.6727, 21.2458) (-23.6567, 21.2271) (-23.6405, 21.2085) (-23.6243, 21.19) (-23.6079, 21.1715) (-23.5913, 21.153) (-23.578, 21.1383) (-23.568, 21.1273) (-23.5613, 21.12) (-23.5579, 21.1163) knots 0 0 0 0 0 0 0.01428571 0.02857143 0.04285714 0.05714286 0.07142857 0.08571429 0.1 0.11428571 0.12857143 0.14285714 0.15714286 0.17142857 0.18571429 0.2 0.21428571 0.22857143 0.24285714 0.25714286 0.27142857 0.28571429 0.3 0.31428571 0.32857143 0.34285714 0.35714286 0.37142857 0.38571429 0.4 0.41428571 0.42857143 0.44285714 0.45714286 0.47142857 0.48571429 0.5 0.51428571 0.52857143 0.54285714 0.55714286 0.57142857 0.58571429 0.6 0.61428571 0.62857143 0.64285714 0.65714286 0.67142857 0.68571429 0.7 0.71428571 0.72857143 0.74285714 0.75714286 0.77142857 0.78571429 0.8 0.81428571 0.82857143 0.84285714 0.85714286 0.87142857 0.88571429 0.9 0.91428571 0.92857143 0.94285714 0.95714286 0.97142857 0.98571429 1 1 1 1 1 1
  arc A18 (-23.5579, 21.1163) -> (-22.9327, 21.2406) centre (-25, 30) ccw
  spline S9 degree 5 poles (-22.9327, 21.2406) (-22.931, 21.2453) (-22.9276, 21.2547) (-22.9225, 21.2687) (-22.9158, 21.2874) (-22.9076, 21.3108) (-22.8996, 21.3341) (-22.8916, 21.3575) (-22.8838, 21.3809) (-22.8762, 21.4042) (-22.8686, 21.4276) (-22.8612, 21.451) (-22.854, 21.4743) (-22.8469, 21.4977) (-22.8399, 21.521) (-22.833, 21.5443) (-22.8264, 21.5677) (-22.8198, 21.591) (-22.8134, 21.6143) (-22.8071, 21.6376) (-22.801, 21.6609) (-22.795, 21.6842) (-22.7892, 21.7075) (-22.7835, 21.7308) (-22.7779, 21.754) (-22.7725, 21.7773) (-22.7673, 21.8005) (-22.7622, 21.8237) (-22.7572, 21.8469) (-22.7524, 21.8701) (-22.7478, 21.8933) (-22.7433, 21.9164) (-22.7389, 21.9395) (-22.7348, 21.9627) (-22.7307, 21.9858) (-22.7269, 22.0088) (-22.7232, 22.0319) (-22.7196, 22.0549) (-22.7162, 22.0779) (-22.713, 22.1009) (-22.71, 22.1239) (-22.7071, 22.1468) (-22.7044, 22.1697) (-22.7018, 22.1926) (-22.6995, 22.2154) (-22.6973, 22.2383) (-22.6953, 22.2611) (-22.6934, 22.2838) (-22.6918, 22.3065) (-22.6903, 22.3292) (-22.689, 22.3519) (-22.6879, 22.3745) (-22.6871, 22.3971) (-22.6864, 22.4196) (-22.6859, 22.4421) (-22.6857, 22.4645) (-22.6856, 22.4869) (-22.6857, 22.5093) (-22.686, 22.5316) (-22.6866, 22.5539) (-22.6874, 22.5761) (-22.6885, 22.5982) (-22.6899, 22.6202) (-22.6917, 22.6422) (-22.6937, 22.6641) (-22.696, 22.6859) (-22.6984, 22.7077) (-22.701, 22.7295) (-22.7038, 22.7511) (-22.707, 22.7727) (-22.7109, 22.794) (-22.7148, 22.8109) (-22.7182, 22.8235) (-22.7207, 22.8318) (-22.722, 22.8359) knots -1 -1 -1 -1 -1 -1 -0.98571429 -0.97142857 -0.95714286 -0.94285714 -0.92857143 -0.91428571 -0.9 -0.88571429 -0.87142857 -0.85714286 -0.84285714 -0.82857143 -0.81428571 -0.8 -0.78571429 -0.77142857 -0.75714286 -0.74285714 -0.72857143 -0.71428571 -0.7 -0.68571429 -0.67142857 -0.65714286 -0.64285714 -0.62857143 -0.61428571 -0.6 -0.58571429 -0.57142857 -0.55714286 -0.54285714 -0.52857143 -0.51428571 -0.5 -0.48571429 -0.47142857 -0.45714286 -0.44285714 -0.42857143 -0.41428571 -0.4 -0.38571429 -0.37142857 -0.35714286 -0.34285714 -0.32857143 -0.31428571 -0.3 -0.28571429 -0.27142857 -0.25714286 -0.24285714 -0.22857143 -0.21428571 -0.2 -0.18571429 -0.17142857 -0.15714286 -0.14285714 -0.12857143 -0.11428571 -0.1 -0.08571429 -0.07142857 -0.05714286 -0.04285714 -0.02857143 -0.01428571 0 0 0 0 0 0
  line L9 (-22.722, 22.8359) -> (-22.8084, 23.1089)
  arc A19 (-22.5157, 23.7247) -> (-22.8084, 23.1089) centre (-22.3317, 23.2598) ccw
  arc A20 (-22.5157, 23.7247) -> (-22.3193, 23.806) centre (-25, 30) ccw
  arc A21 (-21.677, 23.5776) -> (-22.3193, 23.806) centre (-22.1207, 23.3471) ccw
  line L10 (-21.677, 23.5776) -> (-21.545, 23.3234)
  spline S10 degree 5 poles (-21.545, 23.3234) (-21.543, 23.3196) (-21.5389, 23.3119) (-21.5325, 23.3007) (-21.5232, 23.286) (-21.5109, 23.2681) (-21.4979, 23.2506) (-21.4846, 23.2333) (-21.4711, 23.2161) (-21.4574, 23.199) (-21.4435, 23.182) (-21.4295, 23.165) (-21.4152, 23.1482) (-21.4006, 23.1316) (-21.3858, 23.1152) (-21.3706, 23.0989) (-21.3553, 23.0828) (-21.3397, 23.0668) (-21.324, 23.0509) (-21.3081, 23.0351) (-21.292, 23.0195) (-21.2758, 23.0039) (-21.2594, 22.9884) (-21.2428, 22.9731) (-21.2261, 22.9579) (-21.2092, 22.9427) (-21.1921, 22.9277) (-21.1748, 22.9128) (-21.1574, 22.8981) (-21.1399, 22.8834) (-21.1222, 22.8688) (-21.1044, 22.8543) (-21.0864, 22.8399) (-21.0683, 22.8256) (-21.05, 22.8114) (-21.0316, 22.7974) (-21.0131, 22.7834) (-20.9944, 22.7695) (-20.9756, 22.7557) (-20.9567, 22.742) (-20.9377, 22.7285) (-20.9185, 22.715) (-20.8992, 22.7016) (-20.8798, 22.6883) (-20.8602, 22.6751) (-20.8406, 22.662) (-20.8208, 22.649) (-20.8009, 22.6361) (-20.7808, 22.6233) (-20.7607, 22.6106) (-20.7405, 22.598) (-20.7201, 22.5854) (-20.6996, 22.573) (-20.679, 22.5607) (-20.6583, 22.5484) (-20.6375, 22.5363) (-20.6166, 22.5243) (-20.5956, 22.5123) (-20.5744, 22.5004) (-20.5532, 22.4887) (-20.5319, 22.477) (-20.5104, 22.4654) (-20.4889, 22.454) (-20.4672, 22.4426) (-20.4455, 22.4313) (-20.4237, 22.4201) (-20.4017, 22.409) (-20.3797, 22.398) (-20.3575, 22.3871) (-20.3353, 22.3763) (-20.313, 22.3655) (-20.295, 22.357) (-20.2815, 22.3507) (-20.2725, 22.3465) (-20.268, 22.3444) knots 0 0 0 0 0 0 0.01428571 0.02857143 0.04285714 0.05714286 0.07142857 0.08571429 0.1 0.11428571 0.12857143 0.14285714 0.15714286 0.17142857 0.18571429 0.2 0.21428571 0.22857143 0.24285714 0.25714286 0.27142857 0.28571429 0.3 0.31428571 0.32857143 0.34285714 0.35714286 0.37142857 0.38571429 0.4 0.41428571 0.42857143 0.44285714 0.45714286 0.47142857 0.48571429 0.5 0.51428571 0.52857143 0.54285714 0.55714286 0.57142857 0.58571429 0.6 0.61428571 0.62857143 0.64285714 0.65714286 0.67142857 0.68571429 0.7 0.71428571 0.72857143 0.74285714 0.75714286 0.77142857 0.78571429 0.8 0.81428571 0.82857143 0.84285714 0.85714286 0.87142857 0.88571429 0.9 0.91428571 0.92857143 0.94285714 0.95714286 0.97142857 0.98571429 1 1 1 1 1 1
  arc A22 (-20.268, 22.3444) -> (-19.738, 22.6985) centre (-25, 30) ccw
  spline S11 degree 5 poles (-19.738, 22.6985) (-19.7382, 22.7035) (-19.7386, 22.7135) (-19.7393, 22.7283) (-19.7403, 22.7482) (-19.7417, 22.7729) (-19.7432, 22.7976) (-19.7448, 22.8222) (-19.7465, 22.8468) (-19.7484, 22.8713) (-19.7503, 22.8958) (-19.7525, 22.9202) (-19.7547, 22.9445) (-19.7571, 22.9688) (-19.7595, 22.9931) (-19.7622, 23.0172) (-19.7649, 23.0414) (-19.7678, 23.0654) (-19.7708, 23.0894) (-19.7739, 23.1134) (-19.7771, 23.1372) (-19.7805, 23.161) (-19.784, 23.1848) (-19.7877, 23.2084) (-19.7915, 23.2321) (-19.7954, 23.2556) (-19.7994, 23.2791) (-19.8036, 23.3025) (-19.8079, 23.3258) (-19.8123, 23.349) (-19.8169, 23.3722) (-19.8216, 23.3953) (-19.8265, 23.4184) (-19.8314, 23.4413) (-19.8366, 23.4642) (-19.8418, 23.487) (-19.8472, 23.5097) (-19.8528, 23.5324) (-19.8584, 23.5549) (-19.8643, 23.5774) (-19.8702, 23.5998) (-19.8763, 23.6221) (-19.8826, 23.6443) (-19.889, 23.6664) (-19.8956, 23.6884) (-19.9023, 23.7103) (-19.9091, 23.7321) (-19.9162, 23.7539) (-19.9233, 23.7755) (-19.9306, 23.797) (-19.9381, 23.8184) (-19.9458, 23.8397) (-19.9536, 23.8609) (-19.9616, 23.882) (-19.9698, 23.9029) (-19.9782, 23.9238) (-19.9867, 23.9445) (-19.9953, 23.9651) (-20.0041, 23.9856) (-20.0132, 24.006) (-20.0224, 24.0262) (-20.0319, 24.0462) (-20.0417, 24.066) (-20.0517, 24.0856) (-20.062, 24.1051) (-20.0724, 24.1244) (-20.083, 24.1436) (-20.0937, 24.1627) (-20.1046, 24.1816) (-20.1158, 24.2003) (-20.1276, 24.2186) (-20.1376, 24.2327) (-20.1455, 24.243) (-20.151, 24.2497) (-20.1538, 24.253) knots -1 -1 -1 -1 -1 -1 -0.98571429 -0.97142857 -0.95714286 -0.94285714 -0.92857143 -0.91428571 -0.9 -0.88571429 -0.87142857 -0.85714286 -0.84285714 -0.82857143 -0.81428571 -0.8 -0.78571429 -0.77142857 -0.75714286 -0.74285714 -0.72857143 -0.71428571 -0.7 -0.68571429 -0.67142857 -0.65714286 -0.64285714 -0.62857143 -0.61428571 -0.6 -0.58571429 -0.57142857 -0.55714286 -0.54285714 -0.52857143 -0.51428571 -0.5 -0.48571429 -0.47142857 -0.45714286 -0.44285714 -0.42857143 -0.41428571 -0.4 -0.38571429 -0.37142857 -0.35714286 -0.34285714 -0.32857143 -0.31428571 -0.3 -0.28571429 -0.27142857 -0.25714286 -0.24285714 -0.22857143 -0.21428571 -0.2 -0.18571429 -0.17142857 -0.15714286 -0.14285714 -0.12857143 -0.11428571 -0.1 -0.08571429 -0.07142857 -0.05714286 -0.04285714 -0.02857143 -0.01428571 0 0 0 0 0 0
  line L11 (-20.1538, 24.253) -> (-20.3381, 24.4722)
  arc A23 (-20.3033, 25.153) -> (-20.3381, 24.4722) centre (-19.9554, 24.794) ccw
  arc A24 (-20.3033, 25.153) -> (-20.153, 25.3033) centre (-25, 30) ccw
  arc A25 (-19.4722, 25.3381) -> (-20.153, 25.3033) centre (-19.794, 24.9554) ccw
  line L12 (-19.4722, 25.3381) -> (-19.253, 25.1538)
  spline S12 degree 5 poles (-19.253, 25.1538) (-19.2497, 25.151) (-19.243, 25.1455) (-19.2327, 25.1376) (-19.2186, 25.1276) (-19.2003, 25.1158) (-19.1816, 25.1046) (-19.1627, 25.0937) (-19.1436, 25.083) (-19.1244, 25.0724) (-19.1051, 25.062) (-19.0856, 25.0517) (-19.066, 25.0417) (-19.0462, 25.0319) (-19.0262, 25.0224) (-19.006, 25.0132) (-18.9856, 25.0041) (-18.9651, 24.9953) (-18.9445, 24.9867) (-18.9238, 24.9782) (-18.9029, 24.9698) (-18.882, 24.9616) (-18.8609, 24.9536) (-18.8397, 24.9458) (-18.8184, 24.9381) (-18.797, 24.9306) (-18.7755, 24.9233) (-18.7539, 24.9162) (-18.7321, 24.9091) (-18.7103, 24.9023) (-18.6884, 24.8956) (-18.6664, 24.889) (-18.6443, 24.8826) (-18.6221, 24.8763) (-18.5998, 24.8702) (-18.5774, 24.8643) (-18.5549, 24.8584) (-18.5324, 24.8528) (-18.5097, 24.8472) (-18.487, 24.8418) (-18.4642, 24.8366) (-18.4413, 24.8314) (-18.4184, 24.8265) (-18.3953, 24.8216) (-18.3722, 24.8169) (-18.349, 24.8123) (-18.3258, 24.8079) (-18.3025, 24.8036) (-18.2791, 24.7994) (-18.2556, 24.7954) (-18.2321, 24.7915) (-18.2084, 24.7877) (-18.1848, 24.784) (-18.161, 24.7805) (-18.1372, 24.7771) (-18.1134, 24.7739) (-18.0894, 24.7708) (-18.0654, 24.7678) (-18.0414, 24.7649) (-18.0172, 24.7622) (-17.9931, 24.7595) (-17.9688, 24.7571) (-17.9445, 24.7547) (-17.9202, 24.7525) (-17.8958, 24.7503) (-17.8713, 24.7484) (-17.8468, 24.7465) (-17.8222, 24.7448) (-17.7976, 24.7432) (-17.7729, 24.7417) (-17.7482, 24.7403) (-17.7283, 24.7393) (-17.7135, 24.7386) (-17.7035, 24.7382) (-17.6985, 24.738) knots 0 0 0 0 0 0 0.01428571 0.02857143 0.04285714 0.05714286 0.07142857 0.08571429 0.1 0.11428571 0.12857143 0.14285714 0.15714286 0.17142857 0.18571429 0.2 0.21428571 0.22857143 0.24285714 0.25714286 0.27142857 0.28571429 0.3 0.31428571 0.32857143 0.34285714 0.35714286 0.37142857 0.38571429 0.4 0.41428571 0.42857143 0.44285714 0.45714286 0.47142857 0.48571429 0.5 0.51428571 0.52857143 0.54285714 0.55714286 0.57142857 0.58571429 0.6 0.61428571 0.62857143 0.64285714 0.65714286 0.67142857 0.68571429 0.7 0.71428571 0.72857143 0.74285714 0.75714286 0.77142857 0.78571429 0.8 0.81428571 0.82857143 0.84285714 0.85714286 0.87142857 0.88571429 0.9 0.91428571 0.92857143 0.94285714 0.95714286 0.97142857 0.98571429 1 1 1 1 1 1
  arc A26 (-17.6985, 24.738) -> (-17.3444, 25.268) centre (-25, 30) ccw
  spline S13 degree 5 poles (-17.3444, 25.268) (-17.3465, 25.2725) (-17.3507, 25.2815) (-17.357, 25.295) (-17.3655, 25.313) (-17.3763, 25.3353) (-17.3871, 25.3575) (-17.398, 25.3797) (-17.409, 25.4017) (-17.4201, 25.4237) (-17.4313, 25.4455) (-17.4426, 25.4672) (-17.454, 25.4889) (-17.4654, 25.5104) (-17.477, 25.5319) (-17.4887, 25.5532) (-17.5004, 25.5744) (-17.5123, 25.5956) (-17.5243, 25.6166) (-17.5363, 25.6375) (-17.5484, 25.6583) (-17.5607, 25.679) (-17.573, 25.6996) (-17.5854, 25.7201) (-17.598, 25.7405) (-17.6106, 25.7607) (-17.6233, 25.7808) (-17.6361, 25.8009) (-17.649, 25.8208) (-17.662, 25.8406) (-17.6751, 25.8602) (-17.6883, 25.8798) (-17.7016, 25.8992) (-17.715, 25.9185) (-17.7285, 25.9377) (-17.742, 25.9567) (-17.7557, 25.9756) (-17.7695, 25.9944) (-17.7834, 26.0131) (-17.7974, 26.0316) (-17.8114, 26.05) (-17.8256, 26.0683) (-17.8399, 26.0864) (-17.8543, 26.1044) (-17.8688, 26.1222) (-17.8834, 26.1399) (-17.8981, 26.1574) (-17.9128, 26.1748) (-17.9277, 26.1921) (-17.9427, 26.2092) (-17.9579, 26.2261) (-17.9731, 26.2428) (-17.9884, 26.2594) (-18.0039, 26.2758) (-18.0195, 26.292) (-18.0351, 26.3081) (-18.0509, 26.324) (-18.0668, 26.3397) (-18.0828, 26.3553) (-18.0989, 26.3706) (-18.1152, 26.3858) (-18.1316, 26.4006) (-18.1482, 26.4152) (-18.165, 26.4295) (-18.182, 26.4435) (-18.199, 26.4574) (-18.2161, 26.4711) (-18.2333, 26.4846) (-18.2506, 26.4979) (-18.2681, 26.5109) (-18.286, 26.5232) (-18.3007, 26.5325) (-18.3119, 26.5389) (-18.3196, 26.543) (-18.3234, 26.545) knots -1 -1 -1 -1 -1 -1 -0.98571429 -0.97142857 -0.95714286 -0.94285714 -0.92857143 -0.91428571 -0.9 -0.88571429 -0.87142857 -0.85714286 -0.84285714 -0.82857143 -0.81428571 -0.8 -0.78571429 -0.77142857 -0.75714286 -0.74285714 -0.72857143 -0.71428571 -0.7 -0.68571429 -0.67142857 -0.65714286 -0.64285714 -0.62857143 -0.61428571 -0.6 -0.58571429 -0.57142857 -0.55714286 -0.54285714 -0.52857143 -0.51428571 -0.5 -0.48571429 -0.47142857 -0.45714286 -0.44285714 -0.42857143 -0.41428571 -0.4 -0.38571429 -0.37142857 -0.35714286 -0.34285714 -0.32857143 -0.31428571 -0.3 -0.28571429 -0.27142857 -0.25714286 -0.24285714 -0.22857143 -0.21428571 -0.2 -0.18571429 -0.17142857 -0.15714286 -0.14285714 -0.12857143 -0.11428571 -0.1 -0.08571429 -0.07142857 -0.05714286 -0.04285714 -0.02857143 -0.01428571 0 0 0 0 0 0
  line L13 (-18.3234, 26.545) -> (-18.5776, 26.677)
  arc A27 (-18.806, 27.3193) -> (-18.5776, 26.677) centre (-18.3471, 27.1207) ccw
  arc A28 (-18.806, 27.3193) -> (-18.7247, 27.5157) centre (-25, 30) ccw
  arc A29 (-18.1089, 27.8084) -> (-18.7247, 27.5157) centre (-18.2598, 27.3317) ccw
  line L14 (-18.1089, 27.8084) -> (-17.8359, 27.722)
  spline S14 degree 5 poles (-17.8359, 27.722) (-17.8318, 27.7207) (-17.8235, 27.7182) (-17.8109, 27.7148) (-17.794, 27.7109) (-17.7727, 27.707) (-17.7511, 27.7038) (-17.7295, 27.701) (-17.7077, 27.6984) (-17.6859, 27.696) (-17.6641, 27.6937) (-17.6422, 27.6917) (-17.6202, 27.6899) (-17.5982, 27.6885) (-17.5761, 27.6874) (-17.5539, 27.6866) (-17.5316, 27.686) (-17.5093, 27.6857) (-17.4869, 27.6856) (-17.4645, 27.6857) (-17.4421, 27.6859) (-17.4196, 27.6864) (-17.3971, 27.6871) (-17.3745, 27.6879) (-17.3519, 27.689) (-17.3292, 27.6903) (-17.3065, 27.6918) (-17.2838, 27.6934) (-17.2611, 27.6953) (-17.2383, 27.6973) (-17.2154, 27.6995) (-17.1926, 27.7018) (-17.1697, 27.7044) (-17.1468, 27.7071) (-17.1239, 27.71) (-17.1009, 27.713) (-17.0779, 27.7162) (-17.0549, 27.7196) (-17.0319, 27.7232) (-17.0088, 27.7269) (-16.9858, 27.7307) (-16.9627, 27.7348) (-16.9395, 27.7389) (-16.9164, 27.7433) (-16.8933, 27.7478) (-16.8701, 27.7524) (-16.8469, 27.7572) (-16.8237, 27.7622) (-16.8005, 27.7673) (-16.7773, 27.7725) (-16.754, 27.7779) (-16.7308, 27.7835) (-16.7075, 27.7892) (-16.6842, 27.795) (-16.6609, 27.801) (-16.6376, 27.8071) (-16.6143, 27.8134) (-16.591, 27.8198) (-16.5677, 27.8264) (-16.5443, 27.833) (-16.521, 27.8399) (-16.4977, 27.8469) (-16.4743, 27.854) (-16.451, 27.8612) (-16.4276, 27.8686) (-16.4042, 27.8762) (-16.3809, 27.8838) (-16.3575, 27.8916) (-16.3341, 27.8996) (-16.3108, 27.9076) (-16.2874, 27.9158) (-16.2687, 27.9225) (-16.2547, 27.9276) (-16.2453, 27.931) (-16.2406, 27.9327) knots 0 0 0 0 0 0 0.01428571 0.02857143 0.04285714 0.05714286 0.07142857 0.08571429 0.1 0.11428571 0.12857143 0.14285714 0.15714286 0.17142857 0.18571429 0.2 0.21428571 0.22857143 0.24285714 0.25714286 0.27142857 0.28571429 0.3 0.31428571 0.32857143 0.34285714 0.35714286 0.37142857 0.38571429 0.4 0.41428571 0.42857143 0.44285714 0.45714286 0.47142857 0.48571429 0.5 0.51428571 0.52857143 0.54285714 0.55714286 0.57142857 0.58571429 0.6 0.61428571 0.62857143 0.64285714 0.65714286 0.67142857 0.68571429 0.7 0.71428571 0.72857143 0.74285714 0.75714286 0.77142857 0.78571429 0.8 0.81428571 0.82857143 0.84285714 0.85714286 0.87142857 0.88571429 0.9 0.91428571 0.92857143 0.94285714 0.95714286 0.97142857 0.98571429 1 1 1 1 1 1
  arc A30 (-16.2406, 27.9327) -> (-16.1163, 28.5579) centre (-25, 30) ccw